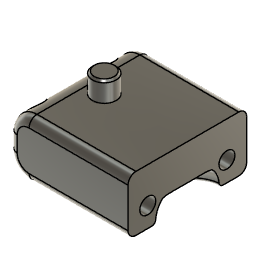
single chanel end bit (spring) (Autodesk Fusion 360 design; units mm, degrees)
Autodesk Fusion 360 part; units mm, degrees
sketch "Sketch1" plane through (0, 0, 0) normal (0, 0, 1) x (1, 0, 0)
  line L0 (0, 0) -> (30, 0)
  line L1 (30, 0) -> (30, 30)
  line L2 (30, 30) -> (0, 30)
  line L3 (0, 30) -> (0, 0)
  dimension "d1" = 30
  dimension "d2" = 30
  constraint horizontal L0
  constraint vertical L1
  constraint horizontal L2
  constraint vertical L3
  constraint coincident L0.start L3.end
  measures "d1" distance of L0.start L0.end
  measures "d2" distance of L0.start L2.end
extrude "Extrude1" add sketch "Sketch1" along normal blind 14
sketch "Sketch2" plane through (0, 0, 0) normal (-1, 0, 0) x (0, -1, 0)
  line L0 (-30, 0) -> (0, 0)
  line L1 (0, 0) -> (0, 14)
  line L2 (0, 14) -> (-30, 14)
  line L3 (-30, 14) -> (-30, 0)
  circle A0 centre (-25, 8.975) radius 2.025
  circle A1 centre (-5, 8.975) radius 2.025
  line L4 (-25, 8.975) -> (-25, 11) construction
  line L5 (-5, 8.975) -> (-5, 11) construction
  dimension "d6" = 4.05
  dimension "d7" = 4.05
  dimension "d29" = 3
  dimension "d30" = 3
  constraint coincident A0.centre L4.start
  constraint coincident A0 L4.end
  constraint parallel L1 L4
  constraint coincident A1.centre L5.start
  constraint coincident A1 L5.end
  constraint parallel L1 L5
  measures "d6" diameter of A0
  measures "d7" diameter of A1
  measures "d29" distance of L2 L4.end
  measures "d30" distance of L2 L5.end
extrude "Extrude2" cut sketch "Sketch2" against normal blind 17 contours A0 | A1
fillet "Fillet1" radius 5 2 edges at (30, 15, 14) (30, 15, 0)
fillet "Fillet2" radius 2 10 edges at (12.5, 30, 0) (28.5355, 30, 1.4645) (30, 30, 7) (28.5355, 30, 12.5355) (12.5, 30, 14) (12.5, 0, 14) (28.5355, 0, 12.5355) (30, 0, 7) (28.5355, 0, 1.4645) (12.5, 0, 0)
sketch "Sketch4" plane through (0, 0, 14) normal (0, 0, 1) x (-1, 0, 0)
  line L0 (0, -2) -> (-25, -2)
  line L1 (-25, -28) -> (0, -28)
  line L2 (0, -28) -> (0, -2)
  circle A0 centre (-30, -24) radius 2
  circle A1 centre (-30, -6) radius 2
  line L3 (-25, -2) -> (-25, -28)
  dimension "d14" = 4
  dimension "d15" = 4
  measures "d14" diameter of A0
  measures "d15" diameter of A1
extrude "Extrude3" cut sketch "Sketch4" against normal blind 15 contours A0 | A1
fillet "Fillet3" radius 1 8 edges at (30, 26, 7) (28, 24, 1) (30, 22, 7) (28, 24, 13) (30, 4, 7) (28, 6, 13) (30, 8, 7) (28, 6, 1)
sketch "Sketch5" plane through (0, 0, 14) normal (0, 0, 1) x (-1, 0, 0)
  line L0 (0, -2) -> (-25, -2)
  line L1 (-25, -28) -> (0, -28)
  line L2 (0, -28) -> (0, -2)
  arc A0 (0, -7) -> (0, -23) centre (1.0714, -15) ccw
  line L3 (-25, -2) -> (-25, -28)
  constraint coincident L2 A0.start
  constraint coincident L2 A0.end
extrude "Extrude4" cut sketch "Sketch5" against normal blind 5 contours L2 A0
fillet "Fillet5" radius 1 1 edges at (7, 15, 14)
chamfer "Chamfer1" distance 2 angle 45 1 edges at (7, 15, 9)
fillet "Fillet6" radius 6 2 edges at (7, 15, 11) (5, 15, 9)
sketch "Sketch6" plane through (0, 0, 0) normal (0, 0, -1) x (1, 0, 0)
  line L0 (25, -2) -> (0, -2)
  line L1 (0, -2) -> (0, -28)
  line L2 (0, -28) -> (25, -28)
  line L3 (25, -28) -> (25, -2)
  circle A0 centre (17, -20) radius 2.5
  line L4 (0, -30) -> (25, -30)
  circle A1 centre (17, -10) radius 2.5
  line L5 (25, 0) -> (0, 0)
  dimension "d31" = 5
  dimension "d32" = 10
  dimension "d33" = 17
  dimension "d34" = 5
  dimension "d35" = 10
  dimension "d36" = 17
  measures "d31" diameter of A0
  measures "d32" distance of A0.centre L4
  measures "d33" distance of L1 A0.centre
  measures "d34" diameter of A1
  measures "d35" distance of A1.centre L5
  measures "d36" distance of L1 A1.centre
sketch "Sketch7" plane through (0, 30, 0) normal (0, 1, 0) x (-1, 0, 0)
  line L0 (-25, 2) -> (0, 2)
  line L1 (0, 2) -> (0, 12)
  line L2 (0, 12) -> (-25, 12)
  arc A0 (-25, 12) -> (-28, 9) centre (-25, 9) ccw
  line L3 (-28, 9) -> (-28, 5)
  arc A1 (-28, 5) -> (-25, 2) centre (-25, 5) ccw
  line L4 (-19.5, 0) -> (-19.5, -1.5)
  line L5 (-18, -1.5) -> (-18, -3)
  line L6 (-19.5, -3) -> (-19.5, -1.5)
  line L7 (-19.5, -3) -> (-19.5, -4.5)
  line L8 (-19.5, -4.5) -> (-18, -3)
  line L9 (-18, -1.5) -> (-19.5, 0)
  dimension "d39" = 1.5
  constraint vertical L4
  constraint vertical L5
  constraint vertical L6
  measures "d39" distance of L4.start L4.end
move_body "Move1" bodies 1 to x (-1, 0, 0) y (0, 1, 0) z (0, 0, -1) at (50, 0, 18)
move_body "Move2" bodies 1 to x (1, 0, 0) y (0, 1, 0) z (0, 0, 1) at (0, 0, -4)
sketch "Sketch8" plane through (0, 0, 14) normal (0, 0, 1) x (-1, 0, 0)
  line L0 (-50, -28) -> (-25, -28)
  line L1 (-25, -28) -> (-25, -2)
  line L2 (-25, -2) -> (-50, -2)
  line L3 (-50, -2) -> (-50, -28)
  circle A0 centre (-29, -15) radius 3
  dimension "d44" = 6
  measures "d44" diameter of A0
extrude "Extrude7" add sketch "Sketch8" along normal blind 5 contours A0
sketch "Sketch9" plane through (0, 30, 0) normal (0, 1, 0) x (-1, 0, 0)
  line L0 (-25, 12) -> (-50, 12)
  line L1 (-50, 12) -> (-50, 2)
  line L2 (-50, 2) -> (-25, 2)
  arc A0 (-25, 2) -> (-22, 5) centre (-25, 5) ccw
  line L3 (-22, 5) -> (-22, 9)
  arc A1 (-22, 9) -> (-25, 12) centre (-25, 9) ccw
  line L4 (-26, 14) -> (-27, 15)
  line L5 (-27, 15) -> (-27, 16)
  line L6 (-27, 16) -> (-26, 17)
  line L7 (-26, 17) -> (-26, 14)
  constraint vertical L5
  constraint parallel L5 L7
extrude "Extrude8" cut sketch "Sketch9" against normal blind 35 contours L4 L5 L6 L7
chamfer "Chamfer2" distance 0.5 angle 45 1 edges at (31.797, 16.0848, 19)
